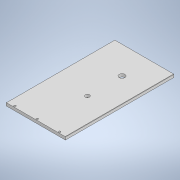
# Autodesk Inventor part: płyta_boczna_obudowy_odbita
Saved by Autodesk Inventor 2020 (Build 240168000, 168)
## iProperties
Created: 2020-08-21
Part Number: płyta_boczna_obudowy_odbita
Material: Generic
Document SubType Name: Modeling
Designer: Hesekiel
Density: 1 g/cm^3
Appearance: Default
Author: Hesekiel
Autodesk Inventor part; units mm, degrees
ref_plane "YZ Plane" through (0, 0, 0) normal (1, 0, 0) x (0, 1, 0)
ref_plane "XZ Plane" through (0, 0, 0) normal (0, 1, 0) x (-1, 0, 0)
ref_plane "XY Plane" through (0, 0, 0) normal (0, 0, 1) x (1, 0, 0)
sketch "Sketch1" plane through (0, 0, 0) normal (0, 1, 0) x (-1, 0, 0)
  line L0 (102.5, 187.5) -> (-102.5, 187.5)
  line L1 (-102.5, 187.5) -> (-102.5, -187.5)
  line L2 (-102.5, -187.5) -> (102.5, -187.5)
  line L3 (102.5, -187.5) -> (102.5, 187.5)
  line L4 (102.5, 187.5) -> (-102.5, -187.5) construction
  line L5 (-102.5, 187.5) -> (102.5, -187.5) construction
  point P0 (0, 0)
  dimension "d0" = 205
  dimension "d1" = 375
  constraints: 12 end point, 2 midpoint, 2 parallel, 1 horizontal, 1 perpendicular
  measures "d0" distance of L2.end L1.end
  measures "d1" distance of L1.end L0.end
extrude "Extrusion1" add sketch "Sketch1" along normal blind 10
fillet "Fillet1" radius 1 2 edges at (102.5, 10, 0) (-102.5, 10, 0)
sketch "Sketch3" plane through (0, 0, 0) normal (0, -1, 0) x (1, 0, 0)
  line L0 (102.5, -187.5) -> (-102.5, -187.5) projected
  line L1 (102.5, 187.5) -> (102.5, -187.5) projected
  line L2 (-102.5, 187.5) -> (102.5, 187.5) projected
  line L3 (-102.5, -187.5) -> (-102.5, 187.5) projected
  line L4 (102.5, 187.5) -> (102.5, -187.5) projected
  line L5 (-102.5, -187.5) -> (-102.5, 187.5) projected
  line L6 (102.5, 187.5) -> (-102.5, 187.5)
  line L7 (-102.5, 187.5) -> (-102.5, 177.5)
  line L8 (-102.5, 177.5) -> (102.5, 177.5)
  line L9 (102.5, 177.5) -> (102.5, 187.5)
  line L10 (102.5, 182.5) -> (77.5, 182.5)
  line L11 (77.5, 182.5) -> (0, 182.5)
  line L12 (0, 182.5) -> (-77.5, 182.5)
  circle A0 centre (77.5, 182.5) radius 3.3
  circle A1 centre (0, 182.5) radius 3.3
  circle A2 centre (-77.5, 182.5) radius 3.3
  point P0 (0, 0)
  dimension "d5" = 10
  dimension "d21" = 25
  dimension "d22" = 77.5
  dimension "d23" = 6.6
  dimension "d24" = 6.6
  dimension "d25" = 6.6
  constraints: 14 end point, 3 centre point, 3 coincident, 3 parallel, 2 horizontal, 2 point on line, 1 midpoint, 1 perpendicular
  measures "d5" distance of L7.end L6.end
  measures "d21" distance of L10.start L10.end
  measures "d22" distance of L11.end L12.end
  measures "d23" diameter of A0
  measures "d24" diameter of A1
  measures "d25" diameter of A2
extrude "Extrusion2" cut sketch "Sketch3" against normal up to surface (10 mm away) contours A2 | A1 L12 L11 | L11 L12 A1 | A0 L11 L10 | L10 L11 A0
sketch "Sketch4" plane through (0, 10, 0) normal (0, 1, 0) x (1, 0, 0)
  line L0 (-101.5, -187.5) -> (-102.5, -187.5) projected
  line L1 (-102.5, -187.5) -> (-18.3, -187.5)
  line L2 (-101.5, -187.5) -> (101.5, -187.5) projected
  line L3 (-18.3, -187.5) -> (-18.3, -27.5)
  circle A0 centre (-18.3, -27.5) radius 7.5
  line L4 (-18.3, -27.5) -> (-18.3, 92.5)
  circle A1 centre (-18.3, 92.5) radius 10
  circle A2 centre (77.5, -182.5) radius 3.3 projected
  circle A3 centre (-77.5, -182.5) radius 3.3 projected
  circle A4 centre (0, -182.5) radius 3.3 projected
  line L5 (-101.5, -187.5) -> (-101.5, 187.5) projected
  line L6 (-101.5, -187.5) -> (101.5, -187.5) projected
  line L7 (101.5, 187.5) -> (101.5, -187.5) projected
  line L8 (101.5, 187.5) -> (-101.5, 187.5) projected
  line L9 (101.5, 187.5) -> (-101.5, 187.5) projected
  line L10 (0, 187.5) -> (0, -187.5)
  circle A5 centre (18.3, -27.5) radius 7.5
  circle A6 centre (18.3, 92.5) radius 10
  point P0 (0, 0)
  dimension "d11" = 84.2
  dimension "d12" = 160
  dimension "d13" = 15
  dimension "d16" = 120
  dimension "d17" = 20
  constraints: 8 end point, 4 centre point, 2 coincident, 2 midpoint, 2 symmetric about line, 1 perpendicular, 1 point on line, 1 vertical, 2 other
  measures "d11" distance of L0.end L1.end
  measures "d12" distance of L1.end L3.end
  measures "d13" diameter of A0
  measures "d16" distance of L4.start L4.end
  measures "d17" diameter of A1
extrude "Extrusion3" cut sketch "Sketch4" against normal up to surface (10 mm away) contours A5 | A6
body "Solid1"
